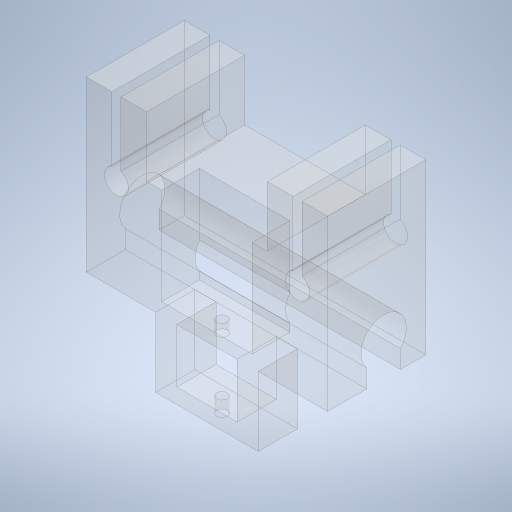
# Autodesk Inventor part: GantryHolder
Saved by Autodesk Inventor 2023 (Build 270158000, 158)
## iProperties
Created: 2022-08-28
Part Number: GantryHolder
Material: PET Plastic
Document SubType Name: Modeling
Designer: Nathann
Density: 1.541 g/cm^3
Appearance: Polycarbonate - Clear
Mass: 135.489 g
Surface Area: 261.555 cm^2
Volume: 87.9228 cm^3
Author: Nathann
Autodesk Inventor part; units mm, degrees
ref_plane "YZ Plane" through (0, 0, 0) normal (1, 0, 0) x (0, 1, 0)
ref_plane "XZ Plane" through (0, 0, 0) normal (0, 1, 0) x (-1, 0, 0)
ref_plane "XY Plane" through (0, 0, 0) normal (0, 0, 1) x (1, 0, 0)
sketch "Sketch1" plane through (0, 0, 0) normal (0, 1, 0) x (-1, 0, 0)
  arc A0 (8.5, 13.7081) -> (11.5, 13.7081) centre (10, 10) ccw
  line L0 (8.5, 20) -> (8.5, 13.7081)
  line L1 (11.5, 20) -> (11.5, 13.7081)
  line L2 (10, 20) -> (10, 18.7339)
  line L3 (20, 20) -> (10, 20)
  line L4 (8.5, 20) -> (0, 20)
  line L5 (0, 20) -> (0, 0)
  line L6 (0, 0) -> (20, 0)
  line L7 (20, 0) -> (20, 20)
  arc A1 (68.5, 13.7081) -> (71.5, 13.7081) centre (70, 10) ccw
  line L8 (68.5, 20) -> (68.5, 13.7081)
  line L9 (71.5, 20) -> (71.5, 13.7081)
  line L10 (70, 20) -> (70, 18.3732)
  line L11 (80, 20) -> (70, 20)
  line L12 (68.5, 20) -> (60.9559, 20)
  line L13 (60.9559, 20) -> (60.9559, 0)
  line L14 (60.9559, 0) -> (80, 0)
  line L15 (80, 0) -> (80, 20)
  line L16 (60.9559, 0) -> (20, 0)
  line L17 (20, 0) -> (20, 20)
  line L18 (20, 20) -> (60.9559, 20)
  line L19 (60.9559, 20) -> (60.9559, 0)
  dimension "d2" = 8
  dimension "d7" = 1.5
  dimension "d8" = 1.5
  dimension "d16" = 10
  dimension "d17" = 8
  dimension "d18" = 1.5
  dimension "d19" = 1.5
  dimension "d20" = 10
  dimension "d22" = 80
  dimension "d23" = 10
  dimension "d24" = 0
  dimension "d25" = 60
  dimension "d26" = 20
  dimension "d27" = 20
  dimension "d28" = 20
  dimension "d29" = 20
  dimension "d30" = 10
  dimension "d31" = 10
  dimension "d32" = 20
  constraints: 40 end point, 6 vertical, 5 perpendicular, 4 parallel, 4 point on circle, 3 point on line, 2 centre point, 1 horizontal
  measures "d2" diameter of A0
  measures "d7" distance between parallel lines of L0 L2
  measures "d8" distance between parallel lines of L1 L2
  measures "d16" horizontal distance of L5.end A0.centre
  measures "d17" diameter of A1
  measures "d18" distance between parallel lines of L8 L10
  measures "d19" distance between parallel lines of L9 L10
  measures "d20" vertical distance of L13.end A1.centre
  measures "d22" distance between parallel lines of L5 L15
  measures "d23" distance from line of L15 A1.centre
  measures "d24" distance between parallel lines of L6 L14
  measures "d25" distance of A0.centre A1.centre
  measures "d26" distance of L14.end L11.start
  measures "d27" distance of L12.end L13.end
  measures "d28" distance of L6.end L3.start
  measures "d29" distance of L4.end L5.end
  measures "d30" distance between parallel lines of L15 L10
  measures "d31" distance between parallel lines of L7 L2
  measures "d32" distance between parallel lines of L16 L18
extrude "Extrusion1" add sketch "Sketch1" along normal blind 36
sketch "Sketch5" plane through (-80, 0, 0) normal (-1, 0, 0) x (0, 0, 1)
  line L0 (20, 0) -> (20, 36) projected
  line L1 (20, 36) -> (-15, 36)
  line L2 (-15, 6) -> (20, 6)
  line L3 (20, 6) -> (20, 36)
  line L4 (-15, 36) -> (-15, 26.6522)
  line L5 (-15, 15.4718) -> (-15, 6)
  line L6 (0, 0) -> (0, 36) projected
  line L7 (0, 0) -> (0, 36) projected
  line L8 (0, 6) -> (0, 36)
  arc A0 (-15, 15.4718) -> (-15, 26.6522) centre (-10, 21.062) ccw
  dimension "d40" = 30
  dimension "d41" = 35
  dimension "d45" = 20
  dimension "d85" = 15
  dimension "d86" = 5
  dimension "d87" = 15
  constraints: 12 end point, 3 parallel, 2 perpendicular, 2 point on circle, 2 point on line, 1 centre point, 1 horizontal, 1 vertical
  measures "d40" distance of L1.end L2.start
  measures "d41" distance of L0.end L1.end
  measures "d45" distance between parallel lines of L0 L6
  measures "d85" diameter of A0
  measures "d86" distance from line of L4 A0.centre
  measures "d87" distance between parallel lines of L6 L5
extrude "Extrusion5" add sketch "Sketch5" against normal blind 80 contours L2 L5 A0 L4 L1 L6
sketch "Sketch13" plane through (0, 36, 0) normal (0, 1, 0) x (1, 0, 0)
  line L0 (-80, -20) -> (-80, 15) projected
  line L1 (-80, -20) -> (-71.5, -20) projected
  line L2 (-71.5, -20) -> (-71.5, -13.7081) projected
  arc A0 (-68.5, -13.7081) -> (-71.5, -13.7081) centre (-70, -10) ccw projected
  line L3 (-68.5, -13.7081) -> (-68.5, -20) projected
  line L4 (-68.5, -20) -> (-11.5, -20) projected
  line L5 (-11.5, -20) -> (-11.5, -13.7081) projected
  arc A1 (-8.5, -13.7081) -> (-11.5, -13.7081) centre (-10, -10) ccw projected
  line L6 (-8.5, -13.7081) -> (-8.5, -20) projected
  line L7 (-8.5, -20) -> (0, -20) projected
  line L8 (0, -20) -> (0, 15) projected
  line L9 (-80, 15) -> (0, 15) projected
  point P0 (0, 0)
extrude "Extrusion11" cut sketch "Sketch13" against normal blind 1
sketch "Sketch16" plane through (-80, 6, -15) normal (0, 0, -1) x (-1, 0, 0)
  line L0 (-80, -6) -> (0, -6) projected
  line L1 (0, 9.4718) -> (-80, 9.4718) projected
  line L2 (-80, -6) -> (0, -6)
  line L3 (0, -6) -> (0, 9.4718)
  line L4 (0, 9.4718) -> (-80, 9.4718)
  line L5 (-80, 9.4718) -> (-80, -6)
  line L6 (0, -6) -> (0, 29) projected
  line L7 (0, 20.6522) -> (-80, 20.6522) projected
  line L8 (0, 29) -> (-80, 29)
  line L9 (-80, 29) -> (-80, 20.6522)
  line L10 (-80, 20.6522) -> (0, 20.6522)
  line L11 (0, 20.6522) -> (0, 29)
  constraints: 16 end point, 4 parallel, 2 horizontal, 2 perpendicular
extrude "Extrusion13" add sketch "Sketch16" along normal blind 6
sketch "Sketch17" plane through (0, 0, 0) normal (0, 0, -1) x (-1, 0, 0)
  line L0 (80, 6) -> (0, 6) projected
  line L1 (0, 0) -> (80, 0) projected
  line L2 (80, 6) -> (0, 6) projected
  line L3 (80, 6) -> (80, 0)
  line L4 (0, 6) -> (0, 0)
  constraints: 4 end point, 1 parallel, 1 perpendicular
extrude "Extrusion14" add sketch "Sketch17" along normal blind 20
sketch "Sketch18" plane through (-68.5, 0, 20) normal (0, 0, 1) x (1, 0, 0)
  line L0 (13.5, 0) -> (43.5, 0)
  line L1 (43.5, 0) -> (43.5, 15)
  line L2 (43.5, 15) -> (13.5, 15)
  line L3 (13.5, 15) -> (13.5, 0)
  line L4 (-11.5, 0) -> (-11.5, 35) projected
  line L5 (0, 0) -> (57, 0) projected
  point P0 (68.5, 0)
  dimension "d107" = 30
  dimension "d108" = 25
  dimension "d109" = 15
  dimension "d110" = 0
  constraints: 8 end point, 2 parallel, 1 horizontal, 1 perpendicular
  measures "d107" distance of L1.end L2.end
  measures "d108" distance between parallel lines of L3 L4
  measures "d109" distance of L2.end L0.start
  measures "d110" distance between parallel lines of L0 L5
extrude "Extrusion15" cut sketch "Sketch18" against normal blind 37
sketch "Sketch19" plane through (0, 0, 0) normal (0, -1, 0) x (1, 0, 0)
  line L0 (-80, -21) -> (0, -21) projected
  line L1 (-30, -21) -> (-23, -21)
  line L2 (-23, -21) -> (-23, -44)
  line L3 (-23, -44) -> (-30, -44)
  line L4 (-30, -44) -> (-30, -21)
  line L5 (-30, -44) -> (-50, -44)
  line L6 (-50, -44) -> (-50, -39)
  line L7 (-50, -39) -> (-30, -39)
  line L8 (-30, -39) -> (-30, -44)
  line L9 (-50, -44) -> (-57, -44)
  line L10 (-57, -44) -> (-57, -21)
  line L11 (-57, -21) -> (-50, -21)
  line L12 (-50, -21) -> (-50, -44)
  line L13 (0, -21) -> (0, 20) projected
  point P0 (0, 0)
  dimension "d113" = 7
  dimension "d114" = 7
  dimension "d115" = 5
  dimension "d116" = 18
  dimension "d117" = 20
  dimension "d118" = 23
  constraints: 24 end point, 6 parallel, 3 horizontal, 3 perpendicular, 2 point on line
  measures "d113" distance between parallel lines of L4 L2
  measures "d114" distance between parallel lines of L10 L12
  measures "d115" distance between parallel lines of L5 L7
  measures "d116" distance between parallel lines of L0 L7
  measures "d117" distance between parallel lines of L12 L4
  measures "d118" distance between parallel lines of L13 L2
extrude "Extrusion16" add sketch "Sketch19" against normal blind 15.5 contours L0 L12 L6 L9 L10 | L0 L2 L3 L4 | L7 L4 L5 L6
sketch "Sketch20" plane through (-23, 0, -44) normal (0, 0, -1) x (-1, 0, 0)
  circle A0 centre (17, 7.5) radius 1.75
  line L0 (34, 0) -> (0, 0) projected
  line L1 (-23, 15.4718) -> (-23, 0) projected
  dimension "d121" = 3.5
  dimension "d122" = 7.5
  dimension "d123" = 40
  constraints: 1 centre point
  measures "d121" diameter of A0
  measures "d122" distance from line of L0 A0.centre
  measures "d123" distance from line of L1 A0.centre
extrude "Extrusion17" cut sketch "Sketch20" against normal blind 80
sketch "Sketch21" plane through (0, 0, 0) normal (0, -1, 0) x (1, 0, 0)
  line L0 (0, -2.5) -> (-80, -2.5) projected
  line L1 (0, -21) -> (-23, -21) projected
  line L2 (0, -21) -> (0, 20) projected
  line L3 (0, 20) -> (-8.5, 20) projected
  line L4 (-8.5, 20) -> (-8.5, 13.7081) projected
  arc A0 (-11.5, 13.7081) -> (-8.5, 13.7081) centre (-10, 10) ccw projected
  line L5 (-11.5, 13.7081) -> (-11.5, 20) projected
  line L6 (-25, 20) -> (-11.5, 20) projected
  line L7 (-25, 20) -> (-25, -17) projected
  line L8 (-25, -17) -> (-55, -17) projected
  line L9 (-55, -17) -> (-55, 20) projected
  line L10 (-68.5, 20) -> (-55, 20) projected
  line L11 (-68.5, 13.7081) -> (-68.5, 20) projected
  arc A1 (-71.5, 13.7081) -> (-68.5, 13.7081) centre (-70, 10) ccw projected
  line L12 (-71.5, 20) -> (-71.5, 13.7081) projected
  line L13 (-80, 20) -> (-71.5, 20) projected
  line L14 (-80, 20) -> (-80, -21) projected
  line L15 (-57, -21) -> (-80, -21) projected
  line L16 (-57, -21) -> (-57, -44) projected
  line L17 (-57, -44) -> (-23, -44) projected
  line L18 (-23, -44) -> (-23, -21) projected
  line L19 (-30, -21) -> (-30, -39) projected
  line L20 (-30, -39) -> (-50, -39) projected
  line L21 (-50, -39) -> (-50, -21) projected
  line L22 (-30, -21) -> (-50, -21) projected
  point P0 (0, 0)
extrude "Extrusion18" cut sketch "Sketch21" against normal blind 2.5 contours L2 L1 L18 L17 L16 L15 L14 L0 L9 L8 L7 | L0 L7 L6 L5 A0 L4 L3 L2 | L0 L14 L13 L12 A1 L11 L10 L9 | L19 L20 L21 L22
sketch "Sketch22" plane through (-68.5, 35, 20) normal (0, 0, 1) x (1, 0, 0)
  line L0 (0, -32.5) -> (13.5, -32.5) projected
  line L1 (13.5, -32.5) -> (13.5, -20) projected
  line L2 (13.5, -20) -> (43.5, -20) projected
  line L3 (43.5, -20) -> (43.5, -32.5) projected
  line L4 (43.5, -32.5) -> (57, -32.5) projected
  line L5 (57, -32.5) -> (57, 0) projected
  line L6 (57, 0) -> (0, 0) projected
  line L7 (0, -32.5) -> (0, 0) projected
  line L8 (60, -32.5) -> (68.5, -32.5) projected
  line L9 (68.5, -32.5) -> (68.5, 0) projected
  line L10 (68.5, 0) -> (60, 0) projected
  line L11 (60, -32.5) -> (60, 0) projected
  line L12 (-11.5, -32.5) -> (-3, -32.5) projected
  line L13 (-3, -32.5) -> (-3, 0) projected
  line L14 (-3, 0) -> (-11.5, 0) projected
  line L15 (-11.5, -32.5) -> (-11.5, 0) projected
  point P0 (68.5, -35)
extrude "Extrusion19" add sketch "Sketch22" along normal blind 15
sketch "Sketch23" plane through (-68.5, 35, 35) normal (0, 0, 1) x (1, 0, 0)
  line L0 (-11.5, 0) -> (68.5, 0) projected
  line L1 (48.5, 0) -> (8.5, 0)
  line L2 (8.5, 0) -> (8.5, -32.5)
  line L3 (8.5, -32.5) -> (48.5, -32.5)
  line L4 (48.5, -32.5) -> (48.5, 0)
  line L5 (68.5, -32.5) -> (68.5, 0) projected
  line L6 (-11.5, 0) -> (-11.5, -32.5) projected
  point P0 (57, 0)
  point P1 (8.5, 0)
  dimension "d130" = 20
  dimension "d131" = 20
  constraints: 8 end point, 2 parallel, 1 horizontal, 1 perpendicular, 1 point on line
  measures "d130" distance between parallel lines of L5 L4
  measures "d131" distance between parallel lines of L6 L2
extrude "Extrusion20" cut sketch "Sketch23" against normal blind 20
equation "\"d2\" = RodDiameter"
equation "\"d17\" = d2"
equation "\"RodDiameter\" = 8"
equation "\"VerticalBearingOD\" = 16"
equation "\"PrintingClearance\" = 0.2"
equation "\"d21\" = 8"
equation "\"TubeID\" = 18"
body "Solid1"
